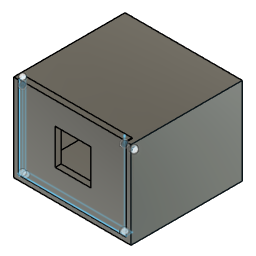
Undercity Card Holder (Autodesk Fusion 360 design; units mm, degrees)
description: Rack; Circular Pitch: 4.12283 mm; Num Teeth: 24; Pressure Angle: 15 deg; Backlash: 0.20 mm;
description: Spur Gear; Module: 1.500000; Num Teeth: 6; Pressure Angle: 20.000000; Backlash: 0.00 mm
Autodesk Fusion 360 part; units mm, degrees
note: some values were not read from the file. Set by a fixed rule: the direction of a hole.
sketch "Sketch1" plane through (0, 0, 0) normal (0, 0, 1) x (1, 0, 0)
  line L0 (-25, 0) -> (-30, 0)
  line L1 (-30, 0) -> (-30, 100)
  line L2 (-30, 100) -> (-25, 100)
  line L3 (-25, 100) -> (-25, 0)
  circle A0 centre (-20, 95) radius 5
  dimension "d1" = 100
  constraint horizontal L0
  constraint vertical L1
  constraint horizontal L2
  constraint vertical L3
  constraint tangent L3 A0
  measures "d1" distance of L0.start L2.end
sketch "Sketch2" plane through (0, 0, 0) normal (0, 0, 1) x (1, 0, 0)
  line L0 (-1.6, 2.5) -> (-1.6, 1.6)
  line L1 (-1.6, 1.6) -> (1.3, 0.6)
  line L2 (1.3, 0.6) -> (1.3, 3.5)
  line L3 (1.3, 3.5) -> (-1.6, 2.5)
  constraint vertical L0
  constraint parallel L0 L2
sketch "Sketch1 (2)" plane through (0, 0, 0) normal (0, 0, 1) x (1, 0, 0) in component "Rack; Circular Pitch: 4.12283 mm; Num Teeth: 24; Pressure Angle: 15 deg; Backlash: 0.20 mm;"
  line L0 (-1.5948, -1.358) -> (0, -0.9307)
  line L1 (0, -0.9307) -> (1.3123, -0.5791)
  line L2 (-1.5948, 1.358) -> (0, 0.9307)
  line L3 (0, 0.9307) -> (1.3123, 0.5791)
  line L4 (1.3123, 0.5791) -> (1.3123, -0.5791)
  line L5 (-1.5948, 1.358) -> (-1.5948, 2.0614)
  line L6 (-1.5948, -1.358) -> (-1.5948, -2.0614)
  line L7 (-1.5948, 2.7648) -> (0, 3.1921)
  line L8 (0, 3.1921) -> (1.3123, 3.5438)
  line L9 (-1.5948, 5.4809) -> (0, 5.0535)
  line L10 (0, 5.0535) -> (1.3123, 4.7019)
  line L11 (1.3123, 4.7019) -> (1.3123, 3.5438)
  line L12 (-1.5948, 5.4809) -> (-1.5948, 6.1842)
  line L13 (-1.5948, 2.7648) -> (-1.5948, 2.0614)
  line L14 (-1.5948, 6.8876) -> (0, 7.315)
  line L15 (0, 7.315) -> (1.3123, 7.6666)
  line L16 (-1.5948, 9.6037) -> (0, 9.1764)
  line L17 (0, 9.1764) -> (1.3123, 8.8247)
  line L18 (1.3123, 8.8247) -> (1.3123, 7.6666)
  line L19 (-1.5948, 9.6037) -> (-1.5948, 10.3071)
  line L20 (-1.5948, 6.8876) -> (-1.5948, 6.1842)
  line L21 (-1.5948, 11.0105) -> (0, 11.4378)
  line L22 (0, 11.4378) -> (1.3123, 11.7894)
  line L23 (-1.5948, 13.7265) -> (0, 13.2992)
  line L24 (0, 13.2992) -> (1.3123, 12.9476)
  line L25 (1.3123, 12.9476) -> (1.3123, 11.7894)
  line L26 (-1.5948, 13.7265) -> (-1.5948, 14.4299)
  line L27 (-1.5948, 11.0105) -> (-1.5948, 10.3071)
  line L28 (-1.5948, 15.1333) -> (0, 15.5606)
  line L29 (0, 15.5606) -> (1.3123, 15.9123)
  line L30 (-1.5948, 17.8494) -> (0, 17.422)
  line L31 (0, 17.422) -> (1.3123, 17.0704)
  line L32 (1.3123, 17.0704) -> (1.3123, 15.9123)
  line L33 (-1.5948, 17.8494) -> (-1.5948, 18.5527)
  line L34 (-1.5948, 15.1333) -> (-1.5948, 14.4299)
  line L35 (-1.5948, 19.2561) -> (0, 19.6834)
  line L36 (0, 19.6834) -> (1.3123, 20.0351)
  line L37 (-1.5948, 21.9722) -> (0, 21.5449)
  line L38 (0, 21.5449) -> (1.3123, 21.1932)
  line L39 (1.3123, 21.1932) -> (1.3123, 20.0351)
  line L40 (-1.5948, 21.9722) -> (-1.5948, 22.6756)
  line L41 (-1.5948, 19.2561) -> (-1.5948, 18.5527)
  line L42 (-1.5948, 23.3789) -> (0, 23.8063)
  line L43 (0, 23.8063) -> (1.3123, 24.1579)
  line L44 (-1.5948, 26.095) -> (0, 25.6677)
  line L45 (0, 25.6677) -> (1.3123, 25.316)
  line L46 (1.3123, 25.316) -> (1.3123, 24.1579)
  line L47 (-1.5948, 26.095) -> (-1.5948, 26.7984)
  line L48 (-1.5948, 23.3789) -> (-1.5948, 22.6756)
  line L49 (-1.5948, 27.5018) -> (0, 27.9291)
  line L50 (0, 27.9291) -> (1.3123, 28.2807)
  line L51 (-1.5948, 30.2178) -> (0, 29.7905)
  line L52 (0, 29.7905) -> (1.3123, 29.4389)
  line L53 (1.3123, 29.4389) -> (1.3123, 28.2807)
  line L54 (-1.5948, 30.2178) -> (-1.5948, 30.9212)
  line L55 (-1.5948, 27.5018) -> (-1.5948, 26.7984)
  line L56 (-1.5948, 31.6246) -> (0, 32.0519)
  line L57 (0, 32.0519) -> (1.3123, 32.4036)
  line L58 (-1.5948, 34.3407) -> (0, 33.9133)
  line L59 (0, 33.9133) -> (1.3123, 33.5617)
  line L60 (1.3123, 33.5617) -> (1.3123, 32.4036)
  line L61 (-1.5948, 34.3407) -> (-1.5948, 35.0441)
  line L62 (-1.5948, 31.6246) -> (-1.5948, 30.9212)
  line L63 (-1.5948, 35.7474) -> (0, 36.1748)
  line L64 (0, 36.1748) -> (1.3123, 36.5264)
  line L65 (-1.5948, 38.4635) -> (0, 38.0362)
  line L66 (0, 38.0362) -> (1.3123, 37.6845)
  line L67 (1.3123, 37.6845) -> (1.3123, 36.5264)
  line L68 (-1.5948, 38.4635) -> (-1.5948, 39.1669)
  line L69 (-1.5948, 35.7474) -> (-1.5948, 35.0441)
  line L70 (-1.5948, 39.8703) -> (0, 40.2976)
  line L71 (0, 40.2976) -> (1.3123, 40.6492)
  line L72 (-1.5948, 42.5863) -> (0, 42.159)
  line L73 (0, 42.159) -> (1.3123, 41.8074)
  line L74 (1.3123, 41.8074) -> (1.3123, 40.6492)
  line L75 (-1.5948, 42.5863) -> (-1.5948, 43.2897)
  line L76 (-1.5948, 39.8703) -> (-1.5948, 39.1669)
  line L77 (-1.5948, 43.9931) -> (0, 44.4204)
  line L78 (0, 44.4204) -> (1.3123, 44.7721)
  line L79 (-1.5948, 46.7092) -> (0, 46.2818)
  line L80 (0, 46.2818) -> (1.3123, 45.9302)
  line L81 (1.3123, 45.9302) -> (1.3123, 44.7721)
  line L82 (-1.5948, 46.7092) -> (-1.5948, 47.4125)
  line L83 (-1.5948, 43.9931) -> (-1.5948, 43.2897)
  line L84 (-1.5948, 48.1159) -> (0, 48.5433)
  line L85 (0, 48.5433) -> (1.3123, 48.8949)
  line L86 (-1.5948, 50.832) -> (0, 50.4047)
  line L87 (0, 50.4047) -> (1.3123, 50.053)
  line L88 (1.3123, 50.053) -> (1.3123, 48.8949)
  line L89 (-1.5948, 50.832) -> (-1.5948, 51.5354)
  line L90 (-1.5948, 48.1159) -> (-1.5948, 47.4125)
  line L91 (-1.5948, 52.2388) -> (0, 52.6661)
  line L92 (0, 52.6661) -> (1.3123, 53.0177)
  line L93 (-1.5948, 54.9548) -> (0, 54.5275)
  line L94 (0, 54.5275) -> (1.3123, 54.1759)
  line L95 (1.3123, 54.1759) -> (1.3123, 53.0177)
  line L96 (-1.5948, 54.9548) -> (-1.5948, 55.6582)
  line L97 (-1.5948, 52.2388) -> (-1.5948, 51.5354)
  line L98 (-1.5948, 56.3616) -> (0, 56.7889)
  line L99 (0, 56.7889) -> (1.3123, 57.1406)
  line L100 (-1.5948, 59.0777) -> (0, 58.6503)
  line L101 (0, 58.6503) -> (1.3123, 58.2987)
  line L102 (1.3123, 58.2987) -> (1.3123, 57.1406)
  line L103 (-1.5948, 59.0777) -> (-1.5948, 59.781)
  line L104 (-1.5948, 56.3616) -> (-1.5948, 55.6582)
  line L105 (-1.5948, 60.4844) -> (0, 60.9117)
  line L106 (0, 60.9117) -> (1.3123, 61.2634)
  line L107 (-1.5948, 63.2005) -> (0, 62.7732)
  line L108 (0, 62.7732) -> (1.3123, 62.4215)
  line L109 (1.3123, 62.4215) -> (1.3123, 61.2634)
  line L110 (-1.5948, 63.2005) -> (-1.5948, 63.9039)
  line L111 (-1.5948, 60.4844) -> (-1.5948, 59.781)
  line L112 (-1.5948, 64.6072) -> (0, 65.0346)
  line L113 (0, 65.0346) -> (1.3123, 65.3862)
  line L114 (-1.5948, 67.3233) -> (0, 66.896)
  line L115 (0, 66.896) -> (1.3123, 66.5443)
  line L116 (1.3123, 66.5443) -> (1.3123, 65.3862)
  line L117 (-1.5948, 67.3233) -> (-1.5948, 68.0267)
  line L118 (-1.5948, 64.6072) -> (-1.5948, 63.9039)
  line L119 (-1.5948, 68.7301) -> (0, 69.1574)
  line L120 (0, 69.1574) -> (1.3123, 69.509)
  line L121 (-1.5948, 71.4461) -> (0, 71.0188)
  line L122 (0, 71.0188) -> (1.3123, 70.6672)
  line L123 (1.3123, 70.6672) -> (1.3123, 69.509)
  line L124 (-1.5948, 71.4461) -> (-1.5948, 72.1495)
  line L125 (-1.5948, 68.7301) -> (-1.5948, 68.0267)
  line L126 (-1.5948, 72.8529) -> (0, 73.2802)
  line L127 (0, 73.2802) -> (1.3123, 73.6319)
  line L128 (-1.5948, 75.569) -> (0, 75.1416)
  line L129 (0, 75.1416) -> (1.3123, 74.79)
  line L130 (1.3123, 74.79) -> (1.3123, 73.6319)
  line L131 (-1.5948, 75.569) -> (-1.5948, 76.2724)
  line L132 (-1.5948, 72.8529) -> (-1.5948, 72.1495)
  line L133 (-1.5948, 76.9757) -> (0, 77.4031)
  line L134 (0, 77.4031) -> (1.3123, 77.7547)
  line L135 (-1.5948, 79.6918) -> (0, 79.2645)
  line L136 (0, 79.2645) -> (1.3123, 78.9128)
  line L137 (1.3123, 78.9128) -> (1.3123, 77.7547)
  line L138 (-1.5948, 79.6918) -> (-1.5948, 80.3952)
  line L139 (-1.5948, 76.9757) -> (-1.5948, 76.2724)
  line L140 (-1.5948, 81.0986) -> (0, 81.5259)
  line L141 (0, 81.5259) -> (1.3123, 81.8775)
  line L142 (-1.5948, 83.8146) -> (0, 83.3873)
  line L143 (0, 83.3873) -> (1.3123, 83.0357)
  line L144 (1.3123, 83.0357) -> (1.3123, 81.8775)
  line L145 (-1.5948, 83.8146) -> (-1.5948, 84.518)
  line L146 (-1.5948, 81.0986) -> (-1.5948, 80.3952)
  line L147 (-1.5948, 85.2214) -> (0, 85.6487)
  line L148 (0, 85.6487) -> (1.3123, 86.0004)
  line L149 (-1.5948, 87.9375) -> (0, 87.5101)
  line L150 (0, 87.5101) -> (1.3123, 87.1585)
  line L151 (1.3123, 87.1585) -> (1.3123, 86.0004)
  line L152 (-1.5948, 87.9375) -> (-1.5948, 88.6408)
  line L153 (-1.5948, 85.2214) -> (-1.5948, 84.518)
  line L154 (-1.5948, 89.3442) -> (0, 89.7716)
  line L155 (0, 89.7716) -> (1.3123, 90.1232)
  line L156 (-1.5948, 92.0603) -> (0, 91.633)
  line L157 (0, 91.633) -> (1.3123, 91.2813)
  line L158 (1.3123, 91.2813) -> (1.3123, 90.1232)
  line L159 (-1.5948, 92.0603) -> (-1.5948, 92.7637)
  line L160 (-1.5948, 89.3442) -> (-1.5948, 88.6408)
  line L161 (-1.5948, 93.4671) -> (0, 93.8944)
  line L162 (0, 93.8944) -> (1.3123, 94.246)
  line L163 (-1.5948, 96.1831) -> (0, 95.7558)
  line L164 (0, 95.7558) -> (1.3123, 95.4042)
  line L165 (1.3123, 95.4042) -> (1.3123, 94.246)
  line L166 (-1.5948, 96.1831) -> (-1.5948, 96.8865)
  line L167 (-1.5948, 93.4671) -> (-1.5948, 92.7637)
  line L168 (-1.5948, 97.5899) -> (0, 98.0172)
  line L169 (0, 98.0172) -> (1.3123, 98.3689)
  line L170 (-1.5948, 100.306) -> (0, 99.8786)
  line L171 (0, 99.8786) -> (1.3123, 99.527)
  line L172 (1.3123, 99.527) -> (1.3123, 98.3689)
  line L173 (-1.5948, 100.306) -> (-1.5948, 101.0093)
  line L174 (-1.5948, 97.5899) -> (-1.5948, 96.8865)
  line L175 (-1.5948, -2.0614) -> (-6.5948, -2.0614)
  line L176 (-6.5948, -2.0614) -> (-6.5948, 96.8865)
  line L177 (-6.5948, 96.8865) -> (-1.5948, 96.8865)
extrude "Extrude1" add sketch "Sketch1 (2)" along normal blind 2.5 and the other way blind 2.5 makes body 1 in component "Rack; Circular Pitch: 4.12283 mm; Num Teeth: 24; Pressure Angle: 15 deg; Backlash: 0.20 mm;"
sketch "Sketch2 (2)" plane through (0, 0, 0) normal (0, 0, 1) x (1, 0, 0) in component "Rack; Circular Pitch: 4.12283 mm; Num Teeth: 24; Pressure Angle: 15 deg; Backlash: 0.20 mm;"
  line L0 (0, 0) -> (0, 94.8251) construction
sketch "Sketch1 (3)" plane through (0, 0, 0) normal (0, 0, 1) x (1, 0, 0) in component "Spur Gear (6 teeth) (2)"
  circle A0 centre (0, 0) radius 2.6492
  circle A1 centre (0, 0) radius 1.5
extrude "Extrude1'" add sketch "Sketch1 (3)" along normal blind 5 separate body makes body 2 in component "Spur Gear (6 teeth) (2)"
sketch "Sketch2 (3)" plane through (0, 0, 0) normal (0, 0, 1) x (1, 0, 0) in component "Spur Gear (6 teeth) (2)"
  spline S0 degree 5 poles (4.0678, -1.1552) (4.0729, -1.1567) (4.0832, -1.1593) (4.0988, -1.1627) (4.1199, -1.1659) (4.1466, -1.1683) (4.1735, -1.1694) (4.2006, -1.1697) (4.2278, -1.1697) (4.2551, -1.1693) (4.2825, -1.1686) (4.31, -1.1674) (4.3375, -1.1657) (4.3651, -1.1633) (4.3929, -1.1604) (4.4207, -1.1568) (4.4486, -1.1527) (4.4765, -1.1482) (4.5045, -1.1432) (4.5325, -1.138) (4.5606, -1.1323) (4.5887, -1.1262) (4.6168, -1.1197) (4.6449, -1.1128) (4.6731, -1.1054) (4.7013, -1.0977) (4.7295, -1.0895) (4.7577, -1.081) (4.7859, -1.0721) (4.8142, -1.0629) (4.8424, -1.0533) (4.8706, -1.0433) (4.8988, -1.0329) (4.927, -1.0222) (4.9552, -1.0112) (4.9834, -0.9998) (5.0115, -0.988) (5.0397, -0.9759) (5.0678, -0.9635) (5.0958, -0.9507) (5.1239, -0.9376) (5.1519, -0.9241) (5.1799, -0.9103) (5.2078, -0.8962) (5.2357, -0.8818) (5.2636, -0.867) (5.2914, -0.8519) (5.3191, -0.8365) (5.3468, -0.8208) (5.3745, -0.8047) (5.4021, -0.7884) (5.4296, -0.7717) (5.4571, -0.7547) (5.4845, -0.7374) (5.5118, -0.7198) (5.5391, -0.7019) (5.5663, -0.6837) (5.5934, -0.6652) (5.6204, -0.6464) (5.6474, -0.6273) (5.6743, -0.6079) (5.7011, -0.5882) (5.7278, -0.5682) (5.7544, -0.5479) (5.7809, -0.5274) (5.8074, -0.5065) (5.8337, -0.4854) (5.86, -0.4639) (5.8861, -0.4422) (5.9121, -0.4202) (5.9381, -0.3979) (5.9588, -0.3799) (5.9742, -0.3662) (5.9845, -0.3571) (5.9896, -0.3525) knots 0 0 0 0 0 0 0.01428571 0.02857143 0.04285714 0.05714286 0.07142857 0.08571429 0.1 0.11428571 0.12857143 0.14285714 0.15714286 0.17142857 0.18571429 0.2 0.21428571 0.22857143 0.24285714 0.25714286 0.27142857 0.28571429 0.3 0.31428571 0.32857143 0.34285714 0.35714286 0.37142857 0.38571429 0.4 0.41428571 0.42857143 0.44285714 0.45714286 0.47142857 0.48571429 0.5 0.51428571 0.52857143 0.54285714 0.55714286 0.57142857 0.58571429 0.6 0.61428571 0.62857143 0.64285714 0.65714286 0.67142857 0.68571429 0.7 0.71428571 0.72857143 0.74285714 0.75714286 0.77142857 0.78571429 0.8 0.81428571 0.82857143 0.84285714 0.85714286 0.87142857 0.88571429 0.9 0.91428571 0.92857143 0.94285714 0.95714286 0.97142857 0.98571429 1 1 1 1 1 1
  spline S1 degree 5 poles (4.0678, 1.1552) (4.0729, 1.1567) (4.0832, 1.1593) (4.0988, 1.1627) (4.1199, 1.1659) (4.1466, 1.1683) (4.1735, 1.1694) (4.2006, 1.1697) (4.2278, 1.1697) (4.2551, 1.1693) (4.2825, 1.1686) (4.31, 1.1674) (4.3375, 1.1657) (4.3651, 1.1633) (4.3929, 1.1604) (4.4207, 1.1568) (4.4486, 1.1527) (4.4765, 1.1482) (4.5045, 1.1432) (4.5325, 1.138) (4.5606, 1.1323) (4.5887, 1.1262) (4.6168, 1.1197) (4.6449, 1.1128) (4.6731, 1.1054) (4.7013, 1.0977) (4.7295, 1.0895) (4.7577, 1.081) (4.7859, 1.0721) (4.8142, 1.0629) (4.8424, 1.0533) (4.8706, 1.0433) (4.8988, 1.0329) (4.927, 1.0222) (4.9552, 1.0112) (4.9834, 0.9998) (5.0115, 0.988) (5.0397, 0.9759) (5.0678, 0.9635) (5.0958, 0.9507) (5.1239, 0.9376) (5.1519, 0.9241) (5.1799, 0.9103) (5.2078, 0.8962) (5.2357, 0.8818) (5.2636, 0.867) (5.2914, 0.8519) (5.3191, 0.8365) (5.3468, 0.8208) (5.3745, 0.8047) (5.4021, 0.7884) (5.4296, 0.7717) (5.4571, 0.7547) (5.4845, 0.7374) (5.5118, 0.7198) (5.5391, 0.7019) (5.5663, 0.6837) (5.5934, 0.6652) (5.6204, 0.6464) (5.6474, 0.6273) (5.6743, 0.6079) (5.7011, 0.5882) (5.7278, 0.5682) (5.7544, 0.5479) (5.7809, 0.5274) (5.8074, 0.5065) (5.8337, 0.4854) (5.86, 0.4639) (5.8861, 0.4422) (5.9121, 0.4202) (5.9381, 0.3979) (5.9588, 0.3799) (5.9742, 0.3662) (5.9845, 0.3571) (5.9896, 0.3525) knots 0 0 0 0 0 0 0.01428571 0.02857143 0.04285714 0.05714286 0.07142857 0.08571429 0.1 0.11428571 0.12857143 0.14285714 0.15714286 0.17142857 0.18571429 0.2 0.21428571 0.22857143 0.24285714 0.25714286 0.27142857 0.28571429 0.3 0.31428571 0.32857143 0.34285714 0.35714286 0.37142857 0.38571429 0.4 0.41428571 0.42857143 0.44285714 0.45714286 0.47142857 0.48571429 0.5 0.51428571 0.52857143 0.54285714 0.55714286 0.57142857 0.58571429 0.6 0.61428571 0.62857143 0.64285714 0.65714286 0.67142857 0.68571429 0.7 0.71428571 0.72857143 0.74285714 0.75714286 0.77142857 0.78571429 0.8 0.81428571 0.82857143 0.84285714 0.85714286 0.87142857 0.88571429 0.9 0.91428571 0.92857143 0.94285714 0.95714286 0.97142857 0.98571429 1 1 1 1 1 1
  arc A0 (5.9896, -0.3525) -> (5.9896, 0.3525) centre (0, 0) ccw
  line L0 (2.5388, -0.7237) -> (4.0678, -1.1552)
  line L1 (2.5388, 0.7237) -> (4.0678, 1.1552)
  line L2 (2.5388, -0.7237) -> (2.5388, 0.7237)
  point P0 (4.1952, -1.1696)
  point P1 (4.3273, -1.1663)
  point P2 (4.4623, -1.1504)
  point P3 (4.5995, -1.1237)
  point P4 (4.7382, -1.0869)
  point P5 (4.878, -1.0405)
  point P6 (5.0186, -0.9849)
  point P7 (5.1594, -0.9204)
  point P8 (5.3001, -0.847)
  point P9 (5.4404, -0.765)
  point P10 (5.5798, -0.6744)
  point P11 (5.7181, -0.5754)
  point P12 (5.8548, -0.4681)
  point P13 (4.1952, 1.1696)
  point P14 (4.3273, 1.1663)
  point P15 (4.4623, 1.1504)
  point P16 (4.5995, 1.1237)
  point P17 (4.7382, 1.0869)
  point P18 (4.878, 1.0405)
  point P19 (5.0186, 0.9849)
  point P20 (5.1594, 0.9204)
  point P21 (5.3001, 0.847)
  point P22 (5.4404, 0.765)
  point P23 (5.5798, 0.6744)
  point P24 (5.7181, 0.5754)
  point P25 (5.8548, 0.4681)
extrude "Extrude2" add sketch "Sketch2 (3)" along normal blind 5 bodies 2 in component "Spur Gear (6 teeth) (2)"
fillet "Fillet1" radius 0.5 2 edges at (2.5477, -0.7262, 2.5) (2.5477, 0.7262, 2.5) on bodies 2 in component "Spur Gear (6 teeth) (2)"
pattern_circular "C-Pattern1" count 6 over 360 about axis through (0, 0, 0) along (0, 0, 1) of "Extrude2", "Fillet1" in component "Spur Gear (6 teeth) (2)"
sketch "Sketch3" plane through (0, 0, 0) normal (0, 0, 1) x (1, 0, 0) in component "Spur Gear (6 teeth) (2)"
  circle A0 centre (0, 0) radius 4.5 construction
sketch "Sketch3 (2)" plane through (0, 0, 0) normal (0, 0, 1) x (1, 0, 0)
  line L0 (25, 0) -> (113.9, 0)
  line L1 (113.9, 0) -> (113.9, 88.9)
  line L2 (113.9, 88.9) -> (25, 88.9)
  line L3 (25, 88.9) -> (25, 0)
  dimension "d86" = 88.9
  dimension "d87" = 88.9
  constraint horizontal L0
  constraint vertical L1
  constraint horizontal L2
  constraint vertical L3
  measures "d86" distance of L0.start L0.end
  measures "d87" distance of L0.start L2.end
extrude "Extrude3" add sketch "Sketch3 (2)" along normal blind 63.5 separate body makes body 3
sketch "Sketch4" plane through (0, 0, 0) normal (0, 1, 0) x (1, 0, 0)
move_body "Move1" bodies 3 to x (1, 0, 0) y (0, 1, 0) z (0, 0, 1) at (-25, 0, 0)
sketch "Sketch5" plane through (0, 0, 0) normal (0, 1, 0) x (1, 0, 0)
  line L0 (1, -1) -> (87, -1)
  line L1 (87, -1) -> (87, -62)
  line L2 (87, -62) -> (1, -62)
  line L3 (1, -62) -> (1, -1)
  constraint horizontal L0
  constraint vertical L1
  constraint horizontal L2
  constraint vertical L3
sketch "Sketch6" plane through (0, 0, 0) normal (0, 1, 0) x (1, 0, 0)
  line L0 (88.9, 0) -> (0, 0)
  line L1 (0, 0) -> (0, -64.5)
  line L2 (0, -64.5) -> (88.9, -64.5)
  line L3 (88.9, -64.5) -> (88.9, 0)
  constraint horizontal L0
  constraint vertical L1
  constraint horizontal L2
  constraint vertical L3
move_face "OffsetFaces1" offset 3 4 faces at (0, 59.2667, 21.1667) (29.6333, 29.6333, 63.5) (29.6333, 29.6333, 0) (88.9, 29.6333, 21.1667) on bodies 3
extrude "Extrude4" cut sketch "Sketch6" along normal blind 86 bodies 3
sketch "Sketch7" plane through (0, 0, 0) normal (0, -1, 0) x (1, 0, 0)
  line L0 (0, 64.5) -> (88.9, 64.5)
  line L1 (88.9, 64.5) -> (88.9, 0)
  line L2 (88.9, 0) -> (0, 0)
  line L3 (0, 0) -> (0, 64.5)
  line L4 (-3, -3) -> (91.9, -3)
  line L5 (91.9, -3) -> (91.9, 66.5)
  line L6 (91.9, 66.5) -> (-3, 66.5)
  line L7 (-3, 66.5) -> (-3, -3)
  line L8 (-3, -3) -> (0, -3)
  line L9 (0, -3) -> (0, 66.5)
  line L10 (0, 66.5) -> (-3, 66.5)
  line L11 (-3, 66.5) -> (-3, -3)
  line L12 (88.9, 66.5) -> (91.9, 66.5)
  line L13 (91.9, 66.5) -> (91.9, -3)
  line L14 (91.9, -3) -> (88.9, -3)
  line L15 (88.9, -3) -> (88.9, 66.5)
  line L16 (91.9, 0) -> (-3, 0)
  line L17 (-3, 0) -> (-3, -3)
  line L18 (-3, -3) -> (91.9, -3)
  line L19 (91.9, -3) -> (91.9, 0)
  constraint horizontal L8
  constraint vertical L9
  constraint horizontal L10
  constraint vertical L11
  constraint coincident L6 L9.end
  constraint coincident L4.start L7.end
  constraint horizontal L12
  constraint vertical L13
  constraint horizontal L14
  constraint vertical L15
  constraint coincident L4.end L5.start
  constraint coincident L6 L12.start
  constraint horizontal L16
  constraint vertical L17
  constraint horizontal L18
  constraint vertical L19
  constraint coincident L13 L16.start
extrude "Extrude5" add sketch "Sketch7" along normal blind 5 contours L3 L6 L7 L9 L10 L11 L16 | L1 L5 L6 L12 L13 L15 L16 | L2 L4 L9 L15 L16 L18 | L4 L7 L8 L9 L11 L16 L17 L18 | L4 L5 L13 L14 L15 L16 L18 L19 bodies 3
sketch "Sketch8" plane through (0, 0, -3) normal (0, 0, -1) x (1, 0, 0)
  line L0 (-3, 5) -> (-3, -88.9)
  line L1 (-3, -88.9) -> (91.9, -88.9)
  line L2 (91.9, -88.9) -> (91.9, 5)
  line L3 (91.9, 5) -> (-3, 5)
  line L4 (-3, -88.9) -> (-3, 5)
  line L5 (-3, 5) -> (-3, -88.9)
  line L6 (91.9, 5) -> (91.9, -88.9)
  line L7 (91.9, -88.9) -> (91.9, 5)
  line L8 (-3, -88.9) -> (-3, 5)
  line L9 (-3, 5) -> (0, 5)
  line L10 (0, 5) -> (0, 0)
  line L11 (0, 0) -> (88.9, 0)
  line L12 (88.9, 0) -> (88.9, 5)
  line L13 (88.9, 5) -> (91.9, 5)
  line L14 (91.9, 5) -> (91.9, -88.9)
  line L15 (91.9, -88.9) -> (-3, -88.9)
move_face "OffsetFaces2" offset 2 4 faces at (59.2667, 59.2667, 66.5) (91.9, 57.6, 20.1667) (-3, 57.6, 43.3333) (28.6333, 57.6, -3) on bodies 3
sketch "Sketch9" plane through (0, 0, 64.5) normal (0, 0, -1) x (1, 0, 0)
  line L0 (88.9, 0) -> (0, 0)
  line L1 (0, 0) -> (0, -86)
  line L2 (0, -86) -> (88.9, -86)
  line L3 (88.9, -86) -> (88.9, 0)
  line L4 (88.9, 0) -> (88.9, -86)
  line L5 (88.9, -86) -> (88.9, 5)
  line L6 (88.9, 5) -> (88.9, 0)
  line L7 (0, 5) -> (0, -86)
  line L8 (0, -86) -> (0, 0)
  line L9 (0, 0) -> (0, 5)
  line L10 (88.9, 5) -> (88.9, -86)
  line L11 (88.9, -86) -> (0, -86)
  line L12 (0, -86) -> (0, 5)
  line L13 (0, 5) -> (88.9, 5)
move_face "OffsetFaces3" offset -1 3 faces at (88.9, 27, 21.5) (0, 27, 21.5) (59.2667, 55.6667, 0) on bodies 3
extrude "Extrude6" add sketch "Sketch7" along normal blind 2 separate body contours L0 L1 L2 L3 L9 L15 L16 makes body 4
move_body "Move2" bodies 4 to x (1, 0, 0) y (0, 1, 0) z (0, 0, 1) at (0, 0, -0.5)
move_body "Move3" bodies 4 to x (1, 0, 0) y (0, 1, 0) z (0, 0, 1) at (0, 2, 0)
sketch "Sketch10" plane through (0, 0, 0) normal (0, 0, 1) x (1, 0, 0)
  line L0 (-1, 0) -> (89.9, 0)
  line L1 (89.9, 0) -> (89.9, -5)
  line L2 (89.9, -5) -> (-1, -5)
  line L3 (-1, -5) -> (-1, 0)
  circle A0 centre (3, -2.5) radius 1.6
  circle A1 centre (86, -2.5) radius 1.6
  dimension "d99" = 3.2
  dimension "d100" = 3.2
  constraint horizontal L0
  constraint vertical L1
  constraint horizontal L2
  constraint vertical L3
  measures "d99" diameter of A0
  measures "d100" diameter of A1
hole "Hole1" at (3, -2.5, 0) direction (0, 0, -1) diameter 3.2 depth 5 tip angle 118 bodies 3
hole "Hole2" at (86, -2.5, 0) direction (0, 0, -1) diameter 3.2 depth 5 tip angle 118 bodies 3
sketch "Sketch11" plane through (0, 0, 0) normal (1, 0, 0) x (0, 1, 0)
  line L0 (-5, -1) -> (0, -1)
  line L1 (0, -1) -> (0, 69)
  line L2 (0, 69) -> (-5, 69)
  line L3 (-5, 69) -> (-5, -1)
  constraint horizontal L0
  constraint vertical L1
  constraint horizontal L2
  constraint vertical L3
extrude "Extrude8" add sketch "Sketch10" along normal blind 70 separate body contours L0 L1 L2 L3 | A0 | A1 makes body 5
hole "Hole3" at (3, -2.5, 0) direction (0, 0, 1) diameter 2.9 depth 30 tip angle 180 bodies 5
hole "Hole4" at (86, -2.5, 0) direction (0, 0, 1) diameter 2.9 depth 30 tip angle 180 bodies 5
sketch "Sketch12" plane through (0, 0, 0) normal (1, 0, 0) x (0, 1, 0)
  line L0 (-2.5, 0) -> (-2.5, 70)
  circle A0 centre (-2.5, 63.9637) radius 1.6
  dimension "d117" = 3.2
  constraint vertical L0
  constraint coincident L0 A0.centre
  measures "d117" diameter of A0
move_body "Move5" bodies 5 to x (1, 0, 0) y (0, 1, 0) z (0, 0, 1) at (0, 0, -1)
hole "Hole5" at (0, -2.5, 63.9637) direction (-1, 0, 0) diameter 2.9 depth 5 tip angle 180 bodies 3 5
hole "Hole6" at (0, -2.5, 63.9637) direction (1, 0, 0) diameter 2.9 depth 30 tip angle 180 bodies 5
hole "Hole7" at (-5, -2.5, 63.9637) direction (1, 0, 0) diameter 3.2 depth 4 tip angle 180 bodies 3
sketch "Sketch13" plane through (93.9, 0, 0) normal (1, 0, 0) x (0, 1, 0)
  line L0 (-5, -5) -> (88.9, -5)
  line L1 (88.9, -5) -> (88.9, 68.5)
  line L2 (88.9, 68.5) -> (-5, 68.5)
  line L3 (-5, 68.5) -> (-5, -5)
  line L4 (-2.5, 0, -7.9) -> (-2.5, 70, -7.9)
  line L5 (-2.5, 70, -7.9) -> (-2.5, 64, -7.9)
  circle A0 through (-0.9, 63.9488, -7.9) (-3.3, 65.3345, -7.9) (-3.3, 62.5632, -7.9)
  dimension "d127" = 3.2
sketch "Sketch14" plane through (93.9, 0, 0) normal (1, 0, 0) x (0, 1, 0)
  circle A0 centre (-2.5, 63.96) radius 1.6
  dimension "d128" = 3.2
  measures "d128" diameter of A0
hole "Hole8" at (93.9, -2.5, 63.96) direction (-1, 0, 0) diameter 3.2 depth 4 tip angle 180 bodies 3
hole "Hole9" at (93.9, -2.5, 63.96) direction (-1, 0, 0) diameter 2.9 depth 30 tip angle 180 bodies 5
sketch "Sketch15" plane through (0, -5, 0) normal (0, -1, 0) x (1, 0, 0)
  line L0 (-1, -1) -> (89.9, -1)
  line L1 (89.9, -1) -> (89.9, 69)
  line L2 (89.9, 69) -> (-1, 69)
  line L3 (-1, 69) -> (-1, -1)
  line L4 (30, 50) -> (60, 50)
  line L5 (60, 50) -> (60, 20)
  line L6 (60, 20) -> (30, 20)
  line L7 (30, 20) -> (30, 50)
  constraint horizontal L4
  constraint vertical L5
  constraint horizontal L6
  constraint vertical L7
extrude "Extrude9" cut sketch "Sketch15" against normal blind 10 contours L4 L5 L6 L7 bodies 5
component "Rack; Circular Pitch: 4.12283 mm; Num Teeth: 24; Pressure Angle: 15 deg; Backlash: 0.20 mm;" placed x (1, 0, 0) y (0, 1, 0) z (0, 0, 1) at (0, 0, 0)
component "Spur Gear (6 teeth) (2)" placed x (1, 0, 0) y (0, 1, 0) z (0, 0, 1) at (0, 0, 0)
hidden bodies 4
